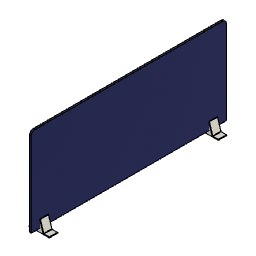
rgiro_sanwa_partition (Autodesk Fusion 360 design; units mm, degrees)
Autodesk Fusion 360 part; units mm, degrees
sketch "Sketch1" plane through (0, 0, 0) normal (0, 0, 1) x (1, 0, 0)
  line L0 (-4.5, -500) -> (4.5, -500)
  line L1 (4.5, -500) -> (4.5, 500)
  line L2 (4.5, 500) -> (-4.5, 500)
  line L3 (-4.5, 500) -> (-4.5, -500)
  line L4 (-4.5, -500) -> (4.5, 500) construction
  line L5 (4.5, -500) -> (-4.5, 500) construction
  dimension "d1" = 1000
  dimension "d2" = 9
  constraint perpendicular L0 L1
  constraint parallel L0 L2
  constraint parallel L1 L3
  constraint horizontal L0
  constraint coincident L4 origin
  constraint coincident L5 origin
  measures "d1" distance of L0.start L2.end
  measures "d2" distance of L0.start L0.end
  measures "d9" distance of L0.start
  measures "d11" distance of L0.start
extrude "Extrude1" add sketch "Sketch1" along normal blind 471 makes body 1
sketch "Sketch3" plane through (4.5, 0, 0) normal (1, 0, 0) x (0, 1, 0)
  line L0 (-500, 0) -> (500, 0)
  line L1 (500, 0) -> (500, 471)
  line L2 (500, 471) -> (-500, 471)
  line L3 (-500, 471) -> (-500, 0)
  line L4 (-500, 0) -> (500, 0)
  line L5 (500, 0) -> (500, 21)
  line L6 (500, 21) -> (-500, 21)
  line L7 (-500, 21) -> (-500, 0)
  dimension "d5" = 21
  constraint horizontal L4
  constraint vertical L5
  constraint horizontal L6
  constraint vertical L7
  constraint coincident L1 L5.end
  constraint coincident L0.start L3.end
  measures "d5" distance of L0.end L5.end
extrude "Extrude2" cut sketch "Sketch3" against normal up to surface (9 mm away) contours L0 L1 L3 L4 L5 L6 L7 bodies 1
fillet "Fillet1" radius 20 2 edges at (0, 500, 471) (0, -500, 471) on bodies 1
sketch "Sketch4" plane through (0, 0, 0) normal (0, 0, 1) x (1, 0, 0)
  line L0 (22.5, -410) -> (-22.5, -410)
  line L1 (-22.5, -410) -> (-22.5, -455)
  line L2 (-22.5, -455) -> (22.5, -455)
  line L3 (22.5, -455) -> (22.5, -410)
  line L4 (22.5, -410) -> (-22.5, -455) construction
  line L5 (-22.5, -410) -> (22.5, -455) construction
  line L6 (22.5, 455) -> (-22.5, 455)
  line L7 (-22.5, 455) -> (-22.5, 410)
  line L8 (-22.5, 410) -> (22.5, 410)
  line L9 (22.5, 410) -> (22.5, 455)
  line L10 (22.5, 455) -> (-22.5, 410) construction
  line L11 (-22.5, 455) -> (22.5, 410) construction
  line L12 (0, -500) -> (0, 500)
  line L13 (-52.5, -455) -> (52.5, -455)
  line L14 (52.5, -455) -> (52.5, -410)
  line L15 (52.5, -410) -> (-52.5, -410)
  line L16 (-52.5, -410) -> (-52.5, -455)
  line L17 (-52.5, -455) -> (52.5, -410) construction
  line L18 (52.5, -455) -> (-52.5, -410) construction
  line L19 (-52.5, 410) -> (52.5, 410)
  line L20 (52.5, 410) -> (52.5, 455)
  line L21 (52.5, 455) -> (-52.5, 455)
  line L22 (-52.5, 455) -> (-52.5, 410)
  line L23 (-52.5, 410) -> (52.5, 455) construction
  line L24 (52.5, 410) -> (-52.5, 455) construction
  point P0 (0, -432.5)
  point P1 (0, 432.5)
  point P2 (0, -432.5)
  point P3 (0, 432.5)
  dimension "d9" = 45
  dimension "d10" = 45
  dimension "d11" = 45
  dimension "d12" = 45
  dimension "d13" = 500
  dimension "d14" = 1000
  dimension "d18" = 105
  dimension "d19" = 105
  constraint perpendicular L0 L1
  constraint parallel L0 L2
  constraint parallel L1 L3
  constraint horizontal L0
  constraint coincident L4 P2
  constraint coincident L5 P2
  constraint perpendicular L6 L7
  constraint parallel L6 L8
  constraint parallel L7 L9
  constraint horizontal L6
  constraint coincident L10 P3
  constraint coincident L11 P3
  constraint equal L0 L6
  constraint equal L3 L9
  constraint vertical L12
  constraint coincident P3 L12
  constraint coincident P2 L12
  constraint coincident origin L12
  constraint perpendicular L13 L14
  constraint parallel L13 L15
  constraint parallel L14 L16
  constraint horizontal L13
  constraint coincident L17 P2
  constraint coincident L18 P2
  constraint coincident P2 P0
  constraint perpendicular L19 L20
  constraint parallel L19 L21
  constraint parallel L20 L22
  constraint horizontal L19
  constraint coincident L23 P3
  constraint coincident L24 P3
  constraint coincident P3 P1
  constraint equal L7 L22
  constraint equal L3 L14
  measures "d9" distance of L6.start L6.end
  measures "d10" distance of L6.start L8.end
  measures "d11" distance of L6 L12.end
  measures "d12" distance of L2 L12.start
  measures "d13" distance of origin L12.start
  measures "d14" distance of L12.start L12.end
  measures "d18" distance of L14.end L15.end
  measures "d19" distance of L20.end L21.end
extrude "Extrude3" add sketch "Sketch4" along normal blind 61 separate body contours L0 L2 L3 L12 L13 L15 | L0 L1 L2 L12 L13 L15 | L6 L8 L9 L12 L19 L21 | L6 L7 L8 L12 L19 L21 makes body 2 at (7.5, -455, 40.6667) makes body 3 at (22.5, 425, 20.3333)
extrude "Extrude4" add sketch "Sketch4" along normal blind 4.5 contours L3 L13 L14 L15 | L1 L13 L15 L16 | L9 L19 L20 L21 | L7 L19 L21 L22 bodies 2 3
sketch "Sketch8" plane through (0, 455, 0) normal (0, 1, 0) x (-1, 0, 0)
  line L0 (-52.5, 0) -> (52.5, 0)
  line L1 (52.5, 0) -> (52.5, 4.5)
  line L2 (52.5, 4.5) -> (22.5, 4.5)
  line L3 (22.5, 4.5) -> (22.5, 61)
  line L4 (22.5, 61) -> (-22.5, 61)
  line L5 (-22.5, 61) -> (-22.5, 4.5)
  line L6 (-22.5, 4.5) -> (-52.5, 4.5)
  line L7 (-52.5, 4.5) -> (-52.5, 0)
  line L8 (4.5, 451) -> (-4.5, 451)
  line L9 (-4.5, 451) -> (-4.5, 21)
  line L10 (-4.5, 21) -> (4.5, 21)
  line L11 (4.5, 21) -> (4.5, 451)
  line L12 (-22.5, 4.5) -> (-22.5, 61)
  line L13 (-4.5, 61) -> (-22.5, 4.5)
  line L14 (4.5, 61) -> (22.5, 61)
  line L15 (22.5, 4.5) -> (4.5, 61)
  constraint coincident L5.end L6.start
  constraint coincident L4.end L5.start
  constraint coincident L4 L13.start
  constraint coincident L9 L13.start
  constraint coincident L4 L14.start
  constraint coincident L11 L14.start
  constraint coincident L3.end L4.start
  constraint coincident L2.end L3.start
extrude "Extrude6" cut sketch "Sketch8" against normal up to surface (910 mm away) contours L4 L5 L12 L13 | L3 L4 L14 L15 bodies 2 3
fillet "Fillet4" radius 2 48 edges at (4.5, -432.5, 61) (-52.5, -432.5, 4.5) (37.5, -410, 4.5) (-13.5, -410, 32.75) (13.5, -410, 32.75) (52.5, -410, 2.25) (-4.5, -432.5, 61) (37.5, -455, 4.5) (-37.5, -455, 4.5) (-37.5, -410, 4.5) (-52.5, -410, 2.25) (0, -410, 0) (0, -455, 0) (52.5, -432.5, 4.5) (-13.5, -455, 32.75) (0, -455, 61) (-52.5, -432.5, 0) (0, -410, 61) (-22.5, -432.5, 4.5) (13.5, -455, 32.75) (22.5, -432.5, 4.5) (52.5, -455, 2.25) (52.5, -432.5, 0) (-52.5, -455, 2.25) (52.5, 410, 2.25) (37.5, 455, 4.5) (0, 410, 0) (37.5, 410, 4.5) (-52.5, 455, 2.25) (52.5, 432.5, 4.5) (-13.5, 410, 32.75) (-52.5, 432.5, 0) (-52.5, 410, 2.25) (0, 455, 61) (-13.5, 455, 32.75) (-22.5, 432.5, 4.5) (0, 410, 61) (52.5, 432.5, 0) (-37.5, 410, 4.5) (22.5, 432.5, 4.5) (-4.5, 432.5, 61) (-52.5, 432.5, 4.5) (4.5, 432.5, 61) (-37.5, 455, 4.5) (52.5, 455, 2.25) (0, 455, 0) (13.5, 455, 32.75) (13.5, 410, 32.75) 20 faces at (1.5, -455, 23.3333) (32.5, -425, 4.5) (-42.5, -440, 4.5) (1.5, -410, 23.3333) (1.5, -440, 61) (-52.5, -425, 1.5) (-16.5, -425, 23.3333) (16.5, -440, 23.3333) (-17.5, -440, 0) (52.5, -440, 1.5) (-16.5, 440, 23.3333) (1.5, 455, 23.3333) (32.5, 440, 4.5) (-32.5, 425, 4.5) (-1.5, 425, 61) (1.5, 410, 23.3333) (52.5, 425, 3) (-17.5, 425, 0) (-52.5, 440, 3) (16.5, 440, 23.3333) on bodies 2 3
